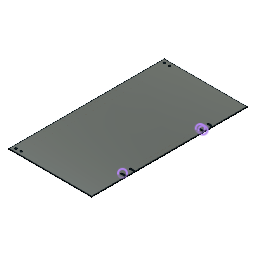
350mm-door-panel-holes (Autodesk Fusion 360 design; units mm, degrees)
Autodesk Fusion 360 part; units mm, degrees
sketch "Sketch1" plane through (0, 0, 0) normal (0, 0, 1) x (1, 0, 0)
  line L0 (-121, 227) -> (121, 227)
  line L1 (121, 227) -> (121, -227)
  line L2 (121, -227) -> (-121, -227)
  line L3 (-121, -227) -> (-121, 227)
  line L4 (-121, 227) -> (121, -227) construction
  line L5 (121, 227) -> (-121, -227) construction
  line L6 (121, -227) -> (121, -113.5) construction
  line L7 (121, -113.5) -> (112, -113.5) construction
  line L8 (112, -113.5) -> (112, -126) construction
  line L9 (112, -113.5) -> (112, -101) construction
  line L10 (0, 0) -> (173.9299, 0) construction
  line L11 (0, 0) -> (-162.2312, 0) construction
  line L12 (-121, -227) -> (-121, -216.6) construction
  line L13 (-121, -216.6) -> (-110.6, -216.6) construction
  circle A0 centre (-110.6, -216.6) radius 2.5
  line L14 (-110.6, -216.6) -> (-95.6, -216.6) construction
  circle A1 centre (-95.6, -216.6) radius 2.5
  line L15 (112, -101) -> (116, -101) construction
  circle A2 centre (116, -101) radius 2
  line L16 (112, -101) -> (108, -101) construction
  circle A3 centre (108, -101) radius 2
  line L17 (107.9064, -99.0022) -> (115.9995, -99)
  line L18 (116, -103) -> (108, -103)
  circle A4 centre (108, -126) radius 2
  line L19 (107.9064, -127.9978) -> (115.9995, -128)
  circle A5 centre (116, -126) radius 2
  line L20 (116, -124) -> (108, -124)
  line L21 (112, 101) -> (108, 101) construction
  line L22 (107.9064, 127.9978) -> (115.9995, 128)
  line L23 (107.9064, 99.0022) -> (115.9995, 99)
  line L24 (116, 103) -> (108, 103)
  line L25 (116, 124) -> (108, 124)
  line L26 (112, 113.5) -> (112, 126) construction
  line L27 (112, 113.5) -> (112, 101) construction
  circle A6 centre (116, 126) radius 2
  line L28 (112, 101) -> (116, 101) construction
  circle A7 centre (108, 126) radius 2
  circle A8 centre (116, 101) radius 2
  circle A9 centre (108, 101) radius 2
  circle A10 centre (-95.6, 216.6) radius 2.5
  circle A11 centre (-110.6, 216.6) radius 2.5
  dimension "d4" = 242
  dimension "d5" = 454
  dimension "d6" = 113.5
  dimension "d9" = 9
  dimension "d10" = 12.5
  dimension "d11" = 12.5
  dimension "d20" = 10.4
  dimension "d21" = 10.4
  dimension "d22" = 5
  dimension "d23" = 15
  dimension "d24" = 5
  dimension "d25" = 4
  dimension "d26" = 4
  dimension "d27" = 4
  dimension "d28" = 4
  constraint horizontal L0
  constraint perpendicular L0 L1
  constraint parallel L0 L2
  constraint parallel L1 L3
  constraint coincident L4 L10.start
  constraint coincident L5 L10.start
  constraint coincident L10.start L11.start
  constraint perpendicular L2 L6
  constraint perpendicular L1 L7
  constraint perpendicular L7 L8
  constraint perpendicular L7 L9
  constraint horizontal L10
  constraint perpendicular L1 L11
  constraint perpendicular L2 L12
  constraint perpendicular L12 L13
  constraint coincident L13.end A0.centre
  constraint parallel L13 L14
  constraint coincident L14.end A1.centre
  constraint perpendicular L9 L15
  constraint coincident L15.end A2.centre
  constraint perpendicular L9 L16
  constraint coincident L16.end A3.centre
  constraint coincident A3 L17.start
  constraint coincident A2 L17.end
  constraint tangent A2 L17
  constraint coincident A2 L18.start
  constraint coincident A3 L18.end
  constraint tangent A3 L18
  constraint parallel L15 L18
  constraint symmetric L7 A2 A5
  constraint symmetric L7 A3 A4
  constraint symmetric L7 L17.start L19.start
  constraint symmetric L7 L17.end L19.end
  constraint symmetric L7 L18.start L20.start
  constraint symmetric L7 L18.end L20.end
  constraint symmetric L7.end L10 L26.start
  constraint symmetric L8.end L10 L26.end
  constraint symmetric L9.end L10 L21.start
  constraint symmetric L10 L15.end L28.end
  constraint symmetric L10 A2 A8
  constraint symmetric L10 L16.end L21.end
  constraint symmetric L10 A3 A9
  constraint symmetric L10 L17.start L23.start
  constraint symmetric L10 L17.end L23.end
  constraint symmetric L10 L18.start L24.start
  constraint symmetric L10 L18.end L24.end
  constraint symmetric L10 A4 A7
  constraint symmetric L10 L19.start L22.start
  constraint symmetric L10 L19.end L22.end
  constraint symmetric L10 A5 A6
  constraint symmetric L10 L20.start L25.start
  constraint symmetric L10 L20.end L25.end
  constraint symmetric L11 A0 A11
  constraint symmetric L11 A1 A10
  measures "d4" distance of L1.end L2.end
  measures "d5" distance of L0.end L1.end
  measures "d6" distance of L1.end L6.end
  measures "d9" distance of L6.end L7.end
  measures "d10" distance of L7.end L8.end
  measures "d11" distance of L7.end L9.end L8.end
  measures "d20" distance of L2.end L12.end
  measures "d21" distance of L12.end L13.end
  measures "d22" diameter of A0
  measures "d23" distance of L13.end L14.end
  measures "d24" diameter of A1
  measures "d25" distance of L9.end L15.end L8.end
  measures "d26" diameter of A2
  measures "d27" distance of L9.end L16.end L8.end
  measures "d28" diameter of A3
extrude "Extrude1" add sketch "Sketch1" along normal blind 2.5 contours L0 L1 L2 L3
sketch "Sketch2" plane through (0, 0, 2.5) normal (0, 0, 1) x (-1, 0, 0)
  arc A0 (-116, -124) -> (-115.9995, -128) centre (-116, -126) ccw
  line L0 (-116, -124) -> (-108, -124)
  arc A1 (-108.0926, -127.9979) -> (-108, -124) centre (-108, -126) ccw
  line L1 (-108.0926, -127.9979) -> (-115.9995, -128)
  line L2 (-108, -103) -> (-116, -103)
  arc A2 (-115.9995, -99) -> (-116, -103) centre (-116, -101) ccw
  line L3 (-115.9995, -99) -> (-108.0926, -99.0021)
  arc A3 (-108, -103) -> (-108.0926, -99.0021) centre (-108, -101) ccw
  circle A4 centre (110.6, -216.6) radius 2.5
  circle A5 centre (95.6, 216.6) radius 2.5
  line L4 (-108, 124) -> (-116, 124)
  arc A6 (-115.9995, 128) -> (-116, 124) centre (-116, 126) ccw
  line L5 (-115.9995, 128) -> (-108.0926, 127.9979)
  arc A7 (-108, 124) -> (-108.0926, 127.9979) centre (-108, 126) ccw
  circle A8 centre (110.6, 216.6) radius 2.5
  circle A9 centre (95.6, -216.6) radius 2.5
  arc A10 (-108.0926, 99.0021) -> (-108, 103) centre (-108, 101) ccw
  line L6 (-108.0926, 99.0021) -> (-115.9995, 99)
  arc A11 (-116, 103) -> (-115.9995, 99) centre (-116, 101) ccw
  line L7 (-116, 103) -> (-108, 103)
  line L8 (121, 227) -> (-121, 227)
  line L9 (-121, 227) -> (-121, -227)
  line L10 (-121, -227) -> (121, -227)
  line L11 (121, -227) -> (121, 227)
equation "doorwidth = 242 mm"
equation "doorheight = 454 mm"
equation "holeradius = 2 mm"
equation "d4 = doorwidth"
equation "d5 = doorheight"
equation "d6 = doorheight / 4"
equation "hingeholestart = 9 mm"
equation "hingeholeseparation = 25 mm"
equation "d9 = hingeholestart"
equation "d10 = hingeholeseparation / 2"
equation "d11 = hingeholeseparation / 2"
equation "hingeholelength = 12 mm"
equation "doorholeseparation = 15 mm"
equation "edgetohandlecenter = 8.05 mm + 2.35 mm"
equation "centertohole = 5.15 mm + 2.35 mm"
equation "d20 = edgetohandlecenter"
equation "d21 = edgetohandlecenter"
equation "d22 = doorholeradius * 2"
equation "d23 = doorholeseparation"
equation "d24 = doorholeradius * 2"
equation "d25 = hingeholelength / 2 - holeradius"
equation "d26 = holeradius * 2"
equation "d27 = hingeholelength / 2 - holeradius"
equation "d28 = holeradius * 2"
equation "doorholeradius = 2.5 mm"
